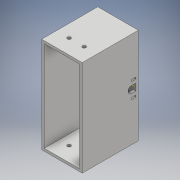
# Autodesk Inventor part: netzteil_case
Saved by Autodesk Inventor 2018 (Build 220112000, 112)
## iProperties
Created: 2018-06-01
Part Number: netzteil_case
Material: Generic
Document SubType Name: Modeling
Designer: bitbots
Density: 1 g/cm^3
Appearance: Default
Author: bitbots
Autodesk Inventor part; units mm, degrees
ref_plane "YZ Plane" through (0, 0, 0) normal (1, 0, 0) x (0, 1, 0)
ref_plane "XZ Plane" through (0, 0, 0) normal (0, 1, 0) x (-1, 0, 0)
ref_plane "XY Plane" through (0, 0, 0) normal (0, 0, 1) x (1, 0, 0)
sketch "Sketch1" plane through (0, 0, 0) normal (0, 1, 0) x (-1, 0, 0)
  line L0 (-20.5, 52.5) -> (20.5, 52.5)
  line L1 (20.5, 52.5) -> (20.5, -52.5)
  line L2 (20.5, -52.5) -> (-20.5, -52.5)
  line L3 (-20.5, -52.5) -> (-20.5, 52.5)
  line L4 (-20.5, 52.5) -> (20.5, -52.5) construction
  line L5 (20.5, 52.5) -> (-20.5, -52.5) construction
  line L6 (-23.5, 55.5) -> (23.5, 55.5)
  line L7 (23.5, 55.5) -> (23.5, -55.5)
  line L8 (23.5, -55.5) -> (-23.5, -55.5)
  line L9 (-23.5, -55.5) -> (-23.5, 55.5)
  line L10 (-23.5, 55.5) -> (23.5, -55.5) construction
  line L11 (23.5, 55.5) -> (-23.5, -55.5) construction
  point P0 (0, 0)
  dimension "d0" = 41
  dimension "d1" = 105
  dimension "d4" = 47
  dimension "d5" = 111
  constraints: 24 end point, 4 midpoint, 4 parallel, 2 horizontal, 2 perpendicular
  measures "d0" distance of L1.end L2.end
  measures "d1" distance of L0.end L1.end
  measures "d4" distance of L7.end L8.end
  measures "d5" distance of L6.end L7.end
extrude "Extrusion1" add sketch "Sketch1" along normal blind 3 contours L0 L1 L2 L3
sketch "Sketch3" plane through (0, 3, 0) normal (0, 1, 0) x (1, 0, 0)
  line L0 (23.5, -55.5) -> (-23.5, -55.5)
  line L1 (-23.5, -55.5) -> (-23.5, 55.5)
  line L2 (-23.5, 55.5) -> (23.5, 55.5)
  line L3 (23.5, 55.5) -> (23.5, -55.5)
  line L4 (23.5, -55.5) -> (-23.5, 55.5) construction
  line L5 (-23.5, -55.5) -> (23.5, 55.5) construction
  line L6 (20.5, 52.5) -> (-20.5, 52.5) projected
  line L7 (20.5, -52.5) -> (-20.5, -52.5)
  line L8 (-20.5, -52.5) -> (-20.5, 52.5)
  line L9 (-20.5, 52.5) -> (20.5, 52.5)
  line L10 (20.5, 52.5) -> (20.5, -52.5)
  line L11 (20.5, -52.5) -> (-20.5, 52.5) construction
  line L12 (-20.5, -52.5) -> (20.5, 52.5) construction
  point P0 (0, 0)
  dimension "d6" = 47
  dimension "d7" = 111
  constraints: 24 end point, 4 midpoint, 4 parallel, 2 horizontal, 2 perpendicular
  measures "d6" distance of L1.end L2.end
  measures "d7" distance of L0.end L1.end
extrude "Extrusion3" add sketch "Sketch3" against normal blind 65
sketch "Sketch4" plane through (23.5, 3, -55.5) normal (0, 0, -1) x (-1, 0, 0)
  line L0 (0, 0) -> (23.5, 0) construction
  line L1 (23.5, 0) -> (23.5, -48) construction
  line L2 (23.5, -48) -> (14.75, -48) construction
  line L3 (23.5, -48) -> (32.25, -48) construction
  circle A0 centre (14.75, -48) radius 2
  circle A1 centre (32.25, -48) radius 2
  point P0 (23.5, -3)
  dimension "d12" = 23.5
  dimension "d13" = 48
  dimension "d14" = 8.75
  dimension "d15" = 8.75
  dimension "d16" = 4
  dimension "d17" = 4
  constraints: 8 end point, 2 centre point, 2 coincident, 2 perpendicular, 1 horizontal, 1 point on line
  measures "d12" distance of L0.start L0.end
  measures "d13" distance of L0.end L1.end
  measures "d14" distance of L1.end L2.end
  measures "d15" distance of L1.end L3.end
  measures "d16" diameter of A0
  measures "d17" diameter of A1
extrude "Extrusion4" cut sketch "Sketch4" against normal blind 3
sketch "Sketch5" plane through (-23.5, 3, 55.5) normal (0, 0, 1) x (1, 0, 0)
  line L0 (47, 0) -> (47, -65) construction
  line L1 (47, 0) -> (23.5, 0) construction
  line L2 (0, 0) -> (47, 0) construction
  line L3 (23.5, 0) -> (23.5, -48) construction
  line L4 (23.5, 0) -> (71.5, 0) construction
  circle A0 centre (32.25, -48) radius 2 projected
  line L5 (23.5, -48) -> (32.25, -48) construction
  circle A1 centre (14.75, -48) radius 2 projected
  line L6 (23.5, -48) -> (14.75, -48) construction
  circle A2 centre (32.25, -48) radius 2 construction
  circle A3 centre (14.75, -48) radius 2 construction
  point P0 (23.5, -3)
  dimension "d20" = 23.5
  dimension "d21" = 48
  dimension "d22" = 90
  constraints: 10 end point, 2 centre point, 2 coincident, 2 concentric, 2 perpendicular, 1 horizontal, 1 midpoint
  measures "d20" distance of L0.start L1.end
  measures "d21" distance of L1.end L3.end
  measures "d22" angle of L3 L4
extrude "Extrusion5" cut sketch "Sketch5" against normal blind 3
sketch "Sketch6" plane through (23.5, 3, 55.5) normal (1, 0, 0) x (0, 0, -1)
  line L0 (111, 0) -> (111, -65) construction
  line L1 (111, 0) -> (55.5, 0) construction
  line L2 (111, 0) -> (0, 0) construction
  line L3 (55.5, 0) -> (51.5, 0) construction
  line L4 (51.5, 0) -> (59.5, 0)
  line L5 (59.5, 0) -> (59.5, -8)
  line L6 (59.5, -8) -> (51.5, -8)
  line L7 (51.5, -8) -> (51.5, 0)
  line L8 (51.5, 0) -> (47.5, 0)
  line L9 (47.5, 0) -> (45.5, 0)
  line L10 (45.5, 0) -> (45.5, -8)
  line L11 (45.5, -8) -> (47.5, -8)
  line L12 (47.5, -8) -> (47.5, 0)
  line L13 (59.5, 0) -> (63.5, 0)
  line L14 (63.5, 0) -> (65.5, 0)
  line L15 (65.5, 0) -> (65.5, -8)
  line L16 (65.5, -8) -> (63.5, -8)
  line L17 (63.5, -8) -> (63.5, 0)
  point P0 (55.5, -3)
  dimension "d25" = 55.5
  dimension "d26" = 4
  dimension "d27" = 8
  dimension "d28" = 8
  dimension "d29" = 4
  dimension "d30" = 2
  dimension "d31" = 4
  dimension "d32" = 2
  dimension "d33" = 8
  constraints: 32 end point, 6 parallel, 3 horizontal, 3 perpendicular, 3 point on line, 1 midpoint
  measures "d25" distance of L0.start L1.end
  measures "d26" distance of L1.end L3.end
  measures "d27" distance of L5.end L6.end
  measures "d28" distance of L4.end L5.end
  measures "d29" distance of L3.end L8.end
  measures "d30" distance of L11.end L10.end
  measures "d31" distance of L4.end L13.end
  measures "d32" distance of L15.end L16.end
  measures "d33" distance of L14.end L15.end
extrude "Extrusion6" cut sketch "Sketch6" against normal blind 3
sketch "Sketch7" plane through (20.5, 3, 55.5) normal (1, 0, 0) x (0, 0, -1)
  point P0 (55.5, -3)
sketch "Sketch8" plane through (20.5, 3, 55.5) normal (1, 0, 0) x (0, 0, -1)
  line L0 (65.5, 0) -> (65.5, -3) projected
  line L1 (63.5, -3) -> (59.5, -3) projected
  line L2 (65.5, 0) -> (63.5, 0)
  line L3 (63.5, 0) -> (63.5, -3)
  line L4 (63.5, -3) -> (65.5, -3)
  line L5 (65.5, -3) -> (65.5, 0)
  line L6 (51.5, 0) -> (59.5, 0) projected
  line L7 (51.5, -3) -> (51.5, 0) projected
  line L8 (59.5, 0) -> (51.5, 0)
  line L9 (51.5, 0) -> (51.5, -3)
  line L10 (51.5, -3) -> (59.5, -3)
  line L11 (59.5, -3) -> (59.5, 0)
  line L12 (51.5, 0) -> (47.5, 0) projected
  line L13 (45.5, -8) -> (45.5, 0) projected
  line L14 (47.5, 0) -> (45.5, 0)
  line L15 (45.5, 0) -> (45.5, -3)
  line L16 (45.5, -3) -> (47.5, -3)
  line L17 (47.5, -3) -> (47.5, 0)
  point P0 (55.5, -3)
  constraints: 24 end point, 6 parallel, 3 horizontal, 3 perpendicular, 2 point on line
extrude "Extrusion7" add sketch "Sketch8" along normal blind 3
sketch "Sketch9" plane through (23.5, 3, 55.5) normal (1, 0, 0) x (0, 0, -1)
  line L0 (59.5, -8) -> (51.5, -8) projected
  circle A0 centre (55.5, -8) radius 4
  point P0 (55.5, -3)
  dimension "d38" = 8
  constraints: 1 centre point, 1 midpoint
  measures "d38" diameter of A0
extrude "Extrusion8" cut sketch "Sketch9" against normal blind 3
sketch "Sketch10" plane through (0, 3, 0) normal (0, 1, 0) x (1, 0, 0)
  line L0 (-23.5, 55.5) -> (23.5, 55.5) projected
  line L1 (0, 55.5) -> (0, 40.5) construction
  line L2 (0, 40.5) -> (0, 35.5) construction
  line L3 (0, 35.5) -> (0, 30.5) construction
  line L4 (0, 30.5) -> (0, 25.5) construction
  line L5 (0, 25.5) -> (0, 20.5) construction
  line L6 (0, 20.5) -> (0, 15.5) construction
  line L7 (0, 15.5) -> (0, 10.5) construction
  line L8 (0, 10.5) -> (0, 5.5) construction
  line L9 (0, 5.5) -> (0, 0.5) construction
  line L10 (-15, 1.5) -> (15, 1.5)
  line L11 (15, 1.5) -> (15, -1.5)
  line L12 (15, -1.5) -> (-15, -1.5)
  line L13 (-15, -1.5) -> (-15, 1.5)
  line L14 (-15, 1.5) -> (15, -1.5) construction
  line L15 (15, 1.5) -> (-15, -1.5) construction
  line L16 (-15, 7) -> (15, 7)
  line L17 (15, 7) -> (15, 4)
  line L18 (15, 4) -> (-15, 4)
  line L19 (-15, 4) -> (-15, 7)
  line L20 (-15, 7) -> (15, 4) construction
  line L21 (15, 7) -> (-15, 4) construction
  line L22 (-15, 12) -> (15, 12)
  line L23 (15, 12) -> (15, 9)
  line L24 (15, 9) -> (-15, 9)
  line L25 (-15, 9) -> (-15, 12)
  line L26 (-15, 12) -> (15, 9) construction
  line L27 (15, 12) -> (-15, 9) construction
  line L28 (-15, 17) -> (15, 17)
  line L29 (15, 17) -> (15, 14)
  line L30 (15, 14) -> (-15, 14)
  line L31 (-15, 14) -> (-15, 17)
  line L32 (-15, 17) -> (15, 14) construction
  line L33 (15, 17) -> (-15, 14) construction
  line L34 (-15, 22) -> (15, 22)
  line L35 (15, 22) -> (15, 19)
  line L36 (15, 19) -> (-15, 19)
  line L37 (-15, 19) -> (-15, 22)
  line L38 (-15, 22) -> (15, 19) construction
  line L39 (15, 22) -> (-15, 19) construction
  line L40 (-15, 27) -> (15, 27)
  line L41 (15, 27) -> (15, 24)
  line L42 (15, 24) -> (-15, 24)
  line L43 (-15, 24) -> (-15, 27)
  line L44 (-15, 27) -> (15, 24) construction
  line L45 (15, 27) -> (-15, 24) construction
  line L46 (-15, 32) -> (15, 32)
  line L47 (15, 32) -> (15, 29)
  line L48 (15, 29) -> (-15, 29)
  line L49 (-15, 29) -> (-15, 32)
  line L50 (-15, 32) -> (15, 29) construction
  line L51 (15, 32) -> (-15, 29) construction
  line L52 (-15, 37) -> (15, 37)
  line L53 (15, 37) -> (15, 34)
  line L54 (15, 34) -> (-15, 34)
  line L55 (-15, 34) -> (-15, 37)
  line L56 (-15, 37) -> (15, 34) construction
  line L57 (15, 37) -> (-15, 34) construction
  line L58 (-15, 42) -> (15, 42)
  line L59 (15, 42) -> (15, 39)
  line L60 (15, 39) -> (-15, 39)
  line L61 (-15, 39) -> (-15, 42)
  line L62 (-15, 42) -> (15, 39) construction
  line L63 (15, 42) -> (-15, 39) construction
  point P0 (0, 0)
  dimension "d41" = 15
  dimension "d42" = 5
  dimension "d43" = 5
  dimension "d44" = 5
  dimension "d45" = 5
  dimension "d46" = 5
  dimension "d47" = 5
  dimension "d48" = 5
  dimension "d49" = 5
  dimension "d50" = 30
  dimension "d51" = 3
  dimension "d52" = 30
  dimension "d53" = 3
  dimension "d54" = 30
  dimension "d55" = 3
  dimension "d56" = 30
  dimension "d57" = 3
  dimension "d58" = 30
  dimension "d59" = 3
  dimension "d60" = 30
  dimension "d61" = 3
  dimension "d62" = 30
  dimension "d63" = 3
  dimension "d64" = 30
  dimension "d65" = 3
  dimension "d66" = 30
  dimension "d67" = 3
  constraints: 126 end point, 19 midpoint, 18 parallel, 9 horizontal, 9 perpendicular, 8 point on line, 1 vertical
  measures "d41" distance of L1.start L1.end
  measures "d42" distance of L1.end L2.end
  measures "d43" distance of L2.end L3.end
  measures "d44" distance of L3.end L4.end
  measures "d45" distance of L4.end L5.end
  measures "d46" distance of L5.end L6.end
  measures "d47" distance of L6.end L7.end
  measures "d48" distance of L7.end L8.end
  measures "d49" distance of L8.end L9.end
  measures "d50" distance of L11.end L12.end
  measures "d51" distance of L10.end L11.end
  measures "d52" distance of L17.end L18.end
  measures "d53" distance of L16.end L17.end
  measures "d54" distance of L23.end L24.end
  measures "d55" distance of L22.end L23.end
  measures "d56" distance of L29.end L30.end
  measures "d57" distance of L28.end L29.end
  measures "d58" distance of L35.end L36.end
  measures "d59" distance of L34.end L35.end
  measures "d60" distance of L41.end L42.end
  measures "d61" distance of L40.end L41.end
  measures "d62" distance of L47.end L48.end
  measures "d63" distance of L46.end L47.end
  measures "d64" distance of L53.end L54.end
  measures "d65" distance of L52.end L53.end
  measures "d66" distance of L59.end L60.end
  measures "d67" distance of L58.end L59.end
extrude "Extrusion9" cut sketch "Sketch10" against normal blind 3
body "Solid1"
